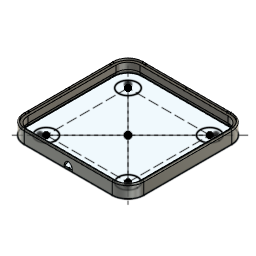
2023_10_02_WoodPlaFootBoard v5 (Autodesk Fusion 360 design; units mm, degrees)
Autodesk Fusion 360 part; units mm, degrees
note: some values were not read from the file. Chosen so that the rebuilt part matches the saved one: which bodies a step acts on; which face or edge a step refers to. Set by a fixed rule: which sketch regions a step uses.
sketch "Sketch1" plane through (0, 0, 0) normal (0, 0, 1) x (1, 0, 0)
  line L0 (65, 65) -> (-65, 65) construction
  line L1 (-65, 65) -> (-65, -65) construction
  line L2 (-65, -65) -> (65, -65) construction
  line L3 (65, -65) -> (65, 65) construction
  line L4 (65, 65) -> (-65, -65) construction
  line L5 (-65, 65) -> (65, -65) construction
  line L6 (70, 95) -> (-70, 95)
  line L7 (-95, 70) -> (-95, -70)
  line L8 (-70, -95) -> (70, -95)
  line L9 (95, -70) -> (95, 70)
  line L10 (95, 95) -> (-95, -95) construction
  line L11 (-95, 95) -> (95, -95) construction
  circle A0 centre (65, 65) radius 14.9
  circle A1 centre (65, -65) radius 14.9
  circle A2 centre (-65, -65) radius 14.9
  circle A3 centre (-65, 65) radius 14.9
  arc A4 (-70, 95) -> (-95, 70) centre (-70, 70) ccw
  arc A5 (95, 70) -> (70, 95) centre (70, 70) ccw
  arc A6 (70, -95) -> (95, -70) centre (70, -70) ccw
  arc A7 (-95, -70) -> (-70, -95) centre (-70, -70) ccw
  dimension "d1" = 130
  dimension "d2" = 130
  dimension "d3" = 190
  dimension "d4" = 190
  dimension "d5" = 29.8
  dimension "d6" = 29.8
  dimension "d7" = 29.8
  dimension "d8" = 29.8
  dimension "d9" = 25
  constraint horizontal L0
  constraint perpendicular L0 L1
  constraint parallel L0 L2
  constraint parallel L1 L3
  constraint coincident L4 origin
  constraint coincident L5 origin
  constraint horizontal L6
  constraint perpendicular L6 L7
  constraint parallel L6 L8
  constraint parallel L7 L9
  constraint coincident L10 origin
  constraint coincident L11 origin
  constraint coincident L0.start L3.end
  constraint coincident L2.end L3.start
  constraint coincident L1.end L2.start
  constraint coincident L0.end L1.start
  constraint coincident L11.start L7
  constraint coincident L11.start L6
  constraint tangent L7 A4
  constraint tangent L6 A4
  constraint coincident L10.start L6
  constraint coincident L10.start L9
  constraint tangent L6 A5
  constraint tangent L9 A5
  constraint equal A4 A5
  constraint coincident L11.end L9
  constraint coincident L11.end L8
  constraint tangent L9 A6
  constraint tangent L8 A6
  constraint equal A4 A6
  constraint coincident L10.end L8
  constraint coincident L10.end L7
  constraint tangent L8 A7
  constraint tangent L7 A7
  constraint equal A4 A7
  measures "d1" distance of L1.end L2.end
  measures "d2" distance of L0.end L1.end
  measures "d3" distance of L10.end L11.end
  measures "d4" distance of L11.start L10.end
  measures "d5" diameter of A0
  measures "d6" diameter of A1
  measures "d7" diameter of A2 L11.start
  measures "d8" diameter of A3 L11.start
  measures "d9" radius of A4
sketch "Sketch2" plane through (0, 0, 0) normal (0, 0, 1) x (1, 0, 0)
  line L0 (-70, -95) -> (70, -95)
  arc A0 (70, -95) -> (95, -70) centre (70, -70) ccw
  line L1 (95, -70) -> (95, 70)
  arc A1 (95, 70) -> (70, 95) centre (70, 70) ccw
  line L2 (70, 95) -> (-70, 95)
  arc A2 (-70, 95) -> (-95, 70) centre (-70, 70) ccw
  line L3 (-95, 70) -> (-95, -70)
  arc A3 (-95, -70) -> (-70, -95) centre (-70, -70) ccw
  line L4 (-93, 70) -> (-93, -70)
  arc A4 (-93, -70) -> (-70, -93) centre (-70, -70) ccw
  line L5 (-70, -93) -> (70, -93)
  arc A5 (70, -93) -> (93, -70) centre (70, -70) ccw
  line L6 (93, -70) -> (93, 70)
  arc A6 (93, 70) -> (70, 93) centre (70, 70) ccw
  line L7 (70, 93) -> (-70, 93)
  arc A7 (-70, 93) -> (-93, 70) centre (-70, 70) ccw
  line L8 (-89, 70) -> (-89, -70)
  arc A8 (-89, -70) -> (-70, -89) centre (-70, -70) ccw
  line L9 (-70, -89) -> (70, -89)
  arc A9 (70, -89) -> (89, -70) centre (70, -70) ccw
  line L10 (89, -70) -> (89, 70)
  arc A10 (89, 70) -> (70, 89) centre (70, 70) ccw
  line L11 (70, 89) -> (-70, 89)
  arc A11 (-70, 89) -> (-89, 70) centre (-70, 70) ccw
  dimension "d14" = 25
  dimension "d19" = -2
  dimension "d24" = -6
  constraint horizontal L2
  constraint perpendicular L2 L3
  constraint parallel L0 L2
  constraint parallel L1 L3
  constraint tangent A2 L3
  constraint tangent L2 A2
  constraint tangent A1 L2
  constraint tangent L1 A1
  constraint equal A1 A2
  constraint tangent A0 L1
  constraint tangent L0 A0
  constraint equal A0 A2
  constraint tangent L0 A3
  constraint tangent L3 A3
  constraint equal A2 A3
  measures "d14" radius of A2
extrude "Extrude1" add sketch "Sketch2" against normal blind 3 contours L0 A0 L1 A1 L2 A2 L3 A3 | L4 A4 L5 A5 L6 A6 L7 A7 | L8 A8 L9 A9 L10 A10 L11 A11 makes body 1
extrude "Extrude2" add sketch "Sketch1" along normal blind 3 separate body makes body 2
move_body "Move1" bodies 1 2 to x (1, 0, 0) y (0, 1, 0) z (0, 0, 1) at (0, 0, 3)
move_body "Move2" bodies 2 to x (1, 0, 0) y (0, 1, 0) z (0, 0, 1) at (0, 0, -3)
move_body "Move3" bodies 2 to x (1, 0, 0) y (0, 1, 0) z (0, 0, 1) at (0, 0, 17)
sketch "Sketch3" plane through (0, 0, 3) normal (0, 0, 1) x (-1, 0, 0)
  arc A0 (95, 70) -> (70, 95) centre (70, 70) ccw
  line L0 (70, 95) -> (-70, 95)
  arc A1 (-70, 95) -> (-95, 70) centre (-70, 70) ccw
  line L1 (-95, 70) -> (-95, -70)
  arc A2 (-95, -70) -> (-70, -95) centre (-70, -70) ccw
  line L2 (-70, -95) -> (70, -95)
  arc A3 (70, -95) -> (95, -70) centre (70, -70) ccw
  line L3 (95, -70) -> (95, 70)
sketch "Sketch4" plane through (0, 0, 0) normal (0, 0, 1) x (1, 0, 0)
extrude "Extrude4" cut sketch "Sketch2" along normal blind 35 contours L0 A0 L1 A1 L2 A2 L3 A3 bodies 1 2
extrude "Extrude5" add sketch "Sketch2" along normal blind 20 separate body contours L0 A0 L1 A1 L2 A2 L3 A3 | L4 A4 L5 A5 L6 A6 L7 A7 makes body 3
combine "Combine1" operation cut target body 3 tool bodies 2 1 keep tools
fillet "Fillet1" radius 4 8 edges at (0, 89, 3) (83.435, 83.435, 3) (89, 0, 3) (83.435, -83.435, 3) (0, -89, 3) (-83.435, -83.435, 3) (-89, 0, 3) (-83.435, 83.435, 3) on bodies 3
sketch "Sketch5" plane through (0, -95, 0) normal (0, -1, 0) x (1, 0, 0)
  line L0 (-70, 0) -> (70, 0)
  line L1 (70, 0) -> (70, 20)
  line L2 (70, 20) -> (-70, 20)
  line L3 (-70, 20) -> (-70, 0)
  ellipse E0 centre (0, 1) end of major axis (0, 11) minor radius 6.6667
  line L4 (0, -9) -> (0, 11)
  line L5 (6.6667, 1) -> (-6.6667, 1)
  constraint coincident E0 L4.start
  constraint coincident E0 L4.end
  constraint coincident E0 L5.start
  constraint coincident E0 L5.end
  constraint vertical L4
extrude "Extrude6" cut sketch "Sketch5" against normal blind 40 contours L0 E0 L4 L5 | L0 E0 L4 | L0 E0 L4 L5 | L0 E0 L4 | E0 L4 L5 | E0 L4 L5 bodies 3
sketch "Sketch6" plane through (0, 0, 0) normal (0, 0, 1) x (1, 0, 0)
  line L0 (70, 93) -> (-70, 93)
  arc A0 (-70, 93) -> (-93, 70) centre (-70, 70) ccw
  line L1 (-93, 70) -> (-93, -70)
  arc A1 (-93, -70) -> (-70, -93) centre (-70, -70) ccw
  line L2 (-70, -93) -> (70, -93)
  arc A2 (70, -93) -> (93, -70) centre (70, -70) ccw
  line L3 (93, -70) -> (93, 70)
  arc A3 (93, 70) -> (70, 93) centre (70, 70) ccw
sketch "Wood Cut Arcade 4 buttons" plane through (0, 0, 20) normal (0, 0, 1) x (-1, 0, 0)
  line L0 (93, -70) -> (93, 70)
  arc A0 (93, 70) -> (70, 93) centre (70, 70) ccw
  line L1 (70, 93) -> (-70, 93)
  arc A1 (-70, 93) -> (-93, 70) centre (-70, 70) ccw
  line L2 (-93, 70) -> (-93, -70)
  arc A2 (-93, -70) -> (-70, -93) centre (-70, -70) ccw
  line L3 (-70, -93) -> (70, -93)
  arc A3 (70, -93) -> (93, -70) centre (70, -70) ccw
  circle A4 centre (65, 65) radius 14.9
  circle A5 centre (-65, 65) radius 14.9
  circle A6 centre (-65, -65) radius 14.9
  circle A7 centre (65, -65) radius 14.9
  arc A8 (93, 70) -> (70, 93) centre (70, 70) ccw
  line L4 (-93, 70) -> (-93, -70)
  arc A9 (-70, 93) -> (-93, 70) centre (-70, 70) ccw
  line L5 (70, 93) -> (-70, 93)
  arc A10 (-93, -70) -> (-70, -93) centre (-70, -70) ccw
  line L6 (93, -70) -> (93, 70)
  line L7 (-70, -93) -> (70, -93)
  arc A11 (70, -93) -> (93, -70) centre (70, -70) ccw
  circle A12 centre (-65, -65) radius 14.9
  line L8 (93, -70) -> (93, 70)
  line L9 (93, -70) -> (93, 70)
  circle A13 centre (-65, 65) radius 14.9
  circle A14 centre (65, 65) radius 14.9
  circle A15 centre (65, -65) radius 14.9
  circle A16 centre (65, -65) radius 14.9
  circle A17 centre (-65, -65) radius 14.9
  circle A18 centre (-65, 65) radius 14.9
  circle A19 centre (65, 65) radius 14.9
  point P0 (-70, 70)
  point P1 (-70, -70)
  point P2 (70, -70)
  point P3 (70, 70)
  point P4 (70, 70)
  point P5 (-70, 70)
  point P6 (70, -70)
  point P7 (-70, -70)
fillet "Fillet2" radius 2 8 edges at (-87.6777, -87.6777, 20) (0, -95, 20) (87.6777, -87.6777, 20) (95, 0, 20) (87.6777, 87.6777, 20) (0, 95, 20) (-87.6777, 87.6777, 20) (-95, 0, 20) on bodies 3
sketch "Sketch8" plane through (0, 0, 0) normal (0, 0, 1) x (1, 0, 0)
  arc A0 (70, -93) -> (93, -70) centre (70, -70) ccw
  line L0 (93, -70) -> (93, 70)
  arc A1 (93, 70) -> (70, 93) centre (70, 70) ccw
  line L1 (70, 93) -> (-70, 93)
  arc A2 (-70, 93) -> (-93, 70) centre (-70, 70) ccw
  line L2 (-93, 70) -> (-93, -70)
  arc A3 (-93, -70) -> (-70, -93) centre (-70, -70) ccw
  line L3 (-70, -93) -> (70, -93)
  arc A4 (70, -92) -> (92, -70) centre (70, -70) ccw
  line L4 (92, -70) -> (92, 70)
  arc A5 (92, 70) -> (70, 92) centre (70, 70) ccw
  line L5 (70, 92) -> (-70, 92)
  arc A6 (-70, 92) -> (-92, 70) centre (-70, 70) ccw
  line L6 (-92, 70) -> (-92, -70)
  arc A7 (-92, -70) -> (-70, -92) centre (-70, -70) ccw
  line L7 (-70, -92) -> (70, -92)
  arc A8 (70, -95) -> (95, -70) centre (70, -70) ccw
  line L8 (95, -70) -> (95, 70)
  arc A9 (95, 70) -> (70, 95) centre (70, 70) ccw
  line L9 (70, 95) -> (-70, 95)
  arc A10 (-70, 95) -> (-95, 70) centre (-70, 70) ccw
  line L10 (-95, 70) -> (-95, -70)
  arc A11 (-95, -70) -> (-70, -95) centre (-70, -70) ccw
  line L11 (-70, -95) -> (70, -95)
  dimension "d33" = -1
  dimension "d34" = 2
extrude "Extrude7" add sketch "Sketch2" sketch "Sketch8" against normal blind 0.2 contours L0 A0 L1 A1 L2 A2 L3 A3 of sketch 2 contours A0 L0 A1 L1 A2 L2 A3 L3 bodies 3
sketch "Sketch9" plane through (0, 0, 0) normal (0, 0, 1) x (1, 0, 0)
sketch "Sketch10" plane through (0, 0, 17) normal (0, 0, 1) x (-1, 0, 0)
  line L0 (89, 70) -> (89, -70)
  arc A0 (70, -89) -> (89, -70) centre (70, -70) ccw
  line L1 (70, -89) -> (-70, -89)
  arc A1 (-89, -70) -> (-70, -89) centre (-70, -70) ccw
  line L2 (-89, -70) -> (-89, 70)
  arc A2 (-70, 89) -> (-89, 70) centre (-70, 70) ccw
  line L3 (-70, 89) -> (70, 89)
  arc A3 (89, 70) -> (70, 89) centre (70, 70) ccw
  line L4 (93, -70) -> (93, 70)
  arc A4 (93, 70) -> (70, 93) centre (70, 70) ccw
  line L5 (70, 93) -> (-70, 93)
  arc A5 (-70, 93) -> (-93, 70) centre (-70, 70) ccw
  line L6 (-93, 70) -> (-93, -70)
  arc A6 (-93, -70) -> (-70, -93) centre (-70, -70) ccw
  line L7 (-70, -93) -> (70, -93)
  arc A7 (70, -93) -> (93, -70) centre (70, -70) ccw
  line L8 (70, 93) -> (-70, 93)
  arc A8 (-70, 93) -> (-93, 70) centre (-70, 70) ccw
  line L9 (-93, 70) -> (-93, -70)
  arc A9 (-93, -70) -> (-70, -93) centre (-70, -70) ccw
  line L10 (-70, -93) -> (70, -93)
  arc A10 (70, -93) -> (93, -70) centre (70, -70) ccw
  line L11 (93, -70) -> (93, 70)
  arc A11 (93, 70) -> (70, 93) centre (70, 70) ccw
  circle A12 centre (93, 0) radius 1
  circle A13 centre (0, 93) radius 1
  circle A14 centre (-93, 0) radius 1
  circle A15 centre (0, -93) radius 1
  point P0 (0, 93)
  point P1 (-93, 0)
  point P2 (0, -93)
  dimension "d37" = 2
  dimension "d39" = 360
  dimension "d41" = 360
  constraint midpoint L11 A12.centre
  measures "d37" diameter of A12
extrude "Extrude8" add sketch "Sketch10" along normal blind 1.5 separate body contours L4 L11 A12 | L7 L10 A15 | L5 L8 A13 | L6 L9 A14 picked at (92.4969, -0.3296) picked at (0.2078, -92.64) picked at (-0.2189, 92.5915) picked at (-92.6667, 0) makes body 4 at (-0.9691, 92.7532, 18) makes body 5 at (0.9691, -92.7532, 18) makes body 6 at (-92.7532, -0.9691, 18) makes body 7 at (92.3572, 0.766, 18)
copy_body "CopyPasteBodies1" bodies 7 makes body 8
move_body "Move4" bodies 8 to x (1, 0, 0) y (0, 1, 0) z (0, 0, 1) at (0, -65, 0)
copy_body "CopyPasteBodies2" bodies 8 makes body 9
move_body "Move5" bodies 9 to x (1, 0, 0) y (0, 1, 0) z (0, 0, 1) at (0, 130, 0)
copy_body "CopyPasteBodies3" bodies 9 7 8 makes body 10 makes body 11 makes body 12
move_body "Move6" bodies 10 11 12 to x (1, 0, 0) y (0, 1, 0) z (0, 0, 1) at (0, 0, -17)
pattern_circular "C-Pattern1" count 4 over 360 about axis through (0, 0, 1.75) along (0, 0, 1) of bodies 8 9 makes body 13 at (64.0012, 92.9502, 18) makes body 14 at (-92.9502, 64.0012, 18) makes body 15 at (-64.0012, -92.9502, 18) makes body 16 at (-65.9988, 92.9502, 18) makes body 17 at (-92.9502, -65.9988, 18) makes body 18 at (65.9988, -92.9502, 18)
combine "Combine2" operation add target body 3 tool bodies 9 4 6 17 5 14 8 7 15 18 13 16
pattern_circular "C-Pattern2" count 4 over 360 about axis through (0, 0, 1.75) along (0, 0, 1) of bodies 12 11 10 makes body 19 at (-65.9988, 92.9502, 1) makes body 20 at (-92.9502, -65.9988, 1) makes body 21 at (65.9988, -92.9502, 1) makes body 22 at (-0.766, 92.3572, 1) makes body 23 at (-92.3572, -0.766, 1) makes body 24 at (0.766, -92.3572, 1) makes body 25 at (64.0012, 92.9502, 1) makes body 26 at (-92.9502, 64.0012, 1) makes body 27 at (-64.0012, -92.9502, 1)
combine "Combine3" operation add target body 3 tool bodies 11 12 10 22 24 23 21 19 20 26 27 25
hidden bodies 1 2
named bodies: "BorderFootBoardPLA"
